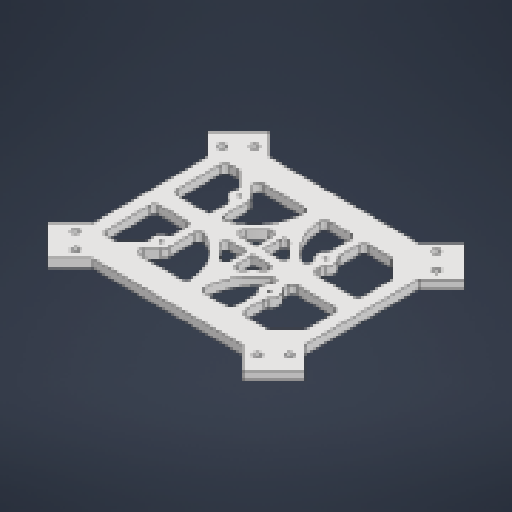
# Autodesk Inventor part: Base
Saved by Autodesk Inventor 2023 (Build 270158000, 158)
## iProperties
Created: 2023-01-21
Part Number: Base
Material: Generic
Document SubType Name: Modeling
Designer: Michael
Density: 1 g/cm^3
Appearance: Default
Author: Michael
Autodesk Inventor part; units mm, degrees
ref_plane "YZ Plane" through (0, 0, 0) normal (1, 0, 0) x (0, 1, 0)
ref_plane "XZ Plane" through (0, 0, 0) normal (0, 1, 0) x (-1, 0, 0)
ref_plane "XY Plane" through (0, 0, 0) normal (0, 0, 1) x (1, 0, 0)
sketch "Sketch1" plane through (0, 0, 0) normal (0, 1, 0) x (-1, 0, 0)
  line L0 (0, 0) -> (152.4, 0)
  line L1 (152.4, 0) -> (152.4, -127)
  line L2 (152.4, -127) -> (0, -127)
  line L3 (0, -127) -> (0, 0)
  circle A0 centre (10.775, -127.8974) radius 2.4765
  circle A1 centre (-0.8987, -116.2224) radius 2.4765
  circle A2 centre (-0.8987, -10.7776) radius 2.4765
  circle A3 centre (10.775, 0.8974) radius 2.4765
  line L4 (76.2, -127) -> (76.2, -50.8058)
  line L5 (152.4, -63.5) -> (91.8437, -63.5)
  line L6 (152.4, 0) -> (0, 0)
  circle A4 centre (10.775, 0.8974) radius 2.4765
  circle A5 centre (-0.8987, -10.7776) radius 2.4765
  line L7 (168.6133, -143.1442) -> (95.3909, -143.1442)
  line L8 (57.0091, -143.1442) -> (6.2091, -143.1442)
  circle A6 centre (153.2987, -10.7776) radius 2.4765
  circle A7 centre (141.625, 0.8974) radius 2.4765
  circle A8 centre (141.625, 0.8974) radius 2.4765
  circle A9 centre (153.2987, -10.7776) radius 2.4765
  line L9 (0, -127) -> (152.4, -127)
  circle A10 centre (-0.8987, -116.2224) radius 2.4765
  circle A11 centre (10.775, -127.8974) radius 2.4765
  circle A12 centre (10.775, -127.8974) radius 2.4765
  circle A13 centre (-0.8987, -116.2224) radius 2.4765
  line L10 (152.4, -127) -> (0, -127)
  line L11 (95.3909, -143.1442) -> (168.6133, -143.1442)
  line L12 (6.2091, -143.1442) -> (57.0091, -143.1442)
  line L13 (6.2832, 16.1645) -> (22.4494, 0)
  line L14 (22.4494, 0) -> (0, -22.4519)
  line L15 (0, -22.4519) -> (-16.1663, -6.2874)
  line L16 (-16.1663, -6.2874) -> (6.2832, 16.1645)
  line L17 (152.4, 0) -> (0, 0)
  line L18 (152.4, -127) -> (152.4, 0)
  circle A14 centre (153.2987, -10.7776) radius 2.4765
  circle A15 centre (141.625, 0.8974) radius 2.4765
  circle A16 centre (141.625, 0.8974) radius 2.4765
  circle A17 centre (153.2987, -10.7776) radius 2.4765
  line L19 (0, 0) -> (152.4, 0)
  line L20 (146.1168, 16.1645) -> (129.9506, 0)
  line L21 (129.9506, 0) -> (152.4, -22.4519)
  line L22 (152.4, -22.4519) -> (168.5663, -6.2874)
  line L23 (168.5663, -6.2874) -> (146.1168, 16.1645)
  line L24 (0, -127) -> (152.4, -127)
  circle A18 centre (-0.8987, -116.2224) radius 2.4765
  circle A19 centre (10.775, -127.8974) radius 2.4765
  circle A20 centre (10.775, -127.8974) radius 2.4765
  circle A21 centre (-0.8987, -116.2224) radius 2.4765
  line L25 (152.4, -127) -> (0, -127)
  circle A22 centre (153.2987, -116.2224) radius 2.4765
  circle A23 centre (153.2987, -116.2224) radius 2.4765
  circle A24 centre (141.625, -127.8974) radius 2.4765
  circle A25 centre (141.625, -127.8974) radius 2.4765
  line L26 (6.2832, -143.1645) -> (22.4494, -127)
  line L27 (22.4494, -127) -> (0, -104.5481)
  line L28 (0, -104.5481) -> (-16.1663, -120.7126)
  line L29 (-16.1663, -120.7126) -> (6.2832, -143.1645)
  line L30 (152.4, -127) -> (0, -127)
  line L31 (0, -127) -> (152.4, -127)
  circle A26 centre (153.2987, -116.2224) radius 2.4765
  circle A27 centre (141.625, -127.8974) radius 2.4765
  circle A28 centre (141.625, -127.8974) radius 2.4765
  circle A29 centre (153.2987, -116.2224) radius 2.4765
  line L32 (129.9506, -127) -> (152.4, -104.5481)
  line L33 (146.1168, -143.1645) -> (129.9506, -127)
  line L34 (152.4, -104.5481) -> (168.5663, -120.7126)
  line L35 (168.5663, -120.7126) -> (146.1168, -143.1645)
  point P0 (76.2, 0)
  point P1 (6.2628, -143.1442)
  point P2 (6.3035, -143.1442)
  point P3 (146.0965, -143.1442)
  point P4 (146.1372, -143.1442)
  dimension "d0" = 152.4
  constraints: 72 end point, 43 symmetric about line, 30 centre point, 4 horizontal, 2 midpoint, 2 parallel, 1 perpendicular, 1 vertical, 46 other
  measures "d0" distance of L1.end L2.end
extrude "Extrusion1" add sketch "Sketch1" along normal blind 6.35 contours L14 L3 A2 L0 A3 | L0 A3 L3 A2 L15 L16 L13 | L0 L21 L1 L32 L2 L27 L3 L14 | L20 L23 L22 L1 A6 L0 A7 | L0 A7 L1 A6 L21 | L27 L2 A0 L3 A1 | L3 A1 L2 A0 L26 L8 L29 L28 | L34 L35 L7 L33 L2 A24 L1 A22 | L1 A22 L2 A24 L32
sketch "Sketch11" plane through (0, 6.35, 0) normal (0, 1, 0) x (1, 0, 0)
  line L0 (-129.9506, 0) -> (-22.4494, 0) projected
  line L1 (-22.4494, 0) -> (-4.4879, -17.9595) projected
  line L2 (-4.4879, -17.9595) -> (17.9615, 4.4923) projected
  line L3 (17.9615, 4.4923) -> (0, 22.4519) projected
  line L4 (0, 22.4519) -> (0, 104.5481) projected
  line L5 (0, 104.5481) -> (17.9615, 122.5077) projected
  line L6 (17.9615, 122.5077) -> (-4.4879, 144.9595) projected
  line L7 (-4.4879, 144.9595) -> (-22.4494, 127) projected
  line L8 (-22.4494, 127) -> (-129.9506, 127) projected
  line L9 (-152.4, 104.5481) -> (-152.4, 22.4519) projected
  circle A0 centre (-10.775, -0.8974) radius 2.4765 projected
  circle A1 centre (0.8987, 10.7776) radius 2.4765 projected
  circle A2 centre (0.8987, 116.2224) radius 2.4765 projected
  circle A3 centre (-10.775, 127.8974) radius 2.4765 projected
  line L10 (-150.1188, 15.875) -> (-4.9505, 15.875)
  line L11 (-76.2, 0) -> (-76.2, 8.5621)
  line L12 (-22.4494, 127) -> (-129.9506, 127) projected
  line L13 (-79.375, 60.1756) -> (-104.775, 60.1756)
  line L14 (-79.375, 60.1756) -> (-79.375, 34.7756)
  arc A4 (-79.375, 34.7756) -> (-104.775, 60.1756) centre (-115.8345, 23.716) ccw
  line L15 (-74.8131, 59.9763) -> (-49.4131, 59.9763)
  line L16 (-74.8131, 59.9763) -> (-74.8131, 34.5763)
  arc A5 (-49.4131, 59.9763) -> (-74.8131, 34.5763) centre (-38.3536, 23.5168) ccw
  line L17 (-116.2036, 57.15) -> (-142.875, 57.15)
  line L18 (-82.272, 21.5362) -> (-82.272, 19.05)
  line L19 (-132.389, 19.05) -> (-142.875, 19.05)
  line L20 (-142.875, 19.05) -> (-142.875, 57.15)
  line L21 (-120.6293, 30.8097) -> (-132.389, 19.05)
  line L22 (-116.2036, 41.4682) -> (-116.2036, 57.15)
  line L23 (-82.272, 19.05) -> (-123.4088, 19.05)
  line L24 (-111.4454, 31.0134) -> (-123.4088, 19.05)
  line L25 (-111.4454, 31.0134) -> (-94.5266, 31.0134) construction
  arc A6 (-111.4454, 31.0134) -> (-109.8536, 35.3392) centre (-116.2025, 35.2196) ccw
  line L26 (-109.8536, 57.0906) -> (-109.8536, 35.3392)
  arc A7 (-82.272, 21.5362) -> (-109.8536, 57.0906) centre (-120.4848, 20.3679) ccw
  line L27 (-71.6381, 21.5362) -> (-71.6381, 18.6974)
  arc A8 (-49.4131, 55.641) -> (-71.6381, 21.5362) centre (-33.4125, 20.9198) ccw
  line L28 (-49.4131, 37.748) -> (-49.4131, 18.6974)
  line L29 (-43.0631, 37.6999) -> (-43.0631, 19.05)
  line L30 (-71.6381, 18.6974) -> (-49.4131, 18.6974)
  line L31 (-49.4131, 48.6912) -> (-49.4131, 55.641)
  arc A9 (-49.4131, 48.6912) -> (-49.4131, 37.748) centre (-46.2025, 43.2196) ccw
  arc A10 (-43.0631, 37.6999) -> (-43.0515, 48.7327) centre (-46.2025, 43.2196) ccw
  line L32 (-43.0631, 19.05) -> (-22.9954, 19.05)
  line L33 (-43.0515, 56.8024) -> (-9.525, 56.8024)
  line L34 (-43.0515, 48.7327) -> (-43.0515, 56.8024)
  line L35 (-9.525, 32.5204) -> (-9.525, 56.8024)
  line L36 (-22.9954, 19.05) -> (-9.525, 32.5204)
  line L37 (-22.9954, 19.05) -> (-3.9454, 19.05) construction
  line L38 (-129.9506, 127) -> (-147.9121, 144.9595) projected
  line L39 (-147.9121, 144.9595) -> (-170.3615, 122.5077) projected
  line L40 (-170.3615, 122.5077) -> (-152.4, 104.5481) projected
  line L41 (-152.4, 22.4519) -> (-170.3615, 4.4923) projected
  line L42 (-170.3615, 4.4923) -> (-147.9121, -17.9595) projected
  line L43 (-147.9121, -17.9595) -> (-129.9506, 0) projected
  line L44 (-76.2, 127) -> (-76.2, 0)
  line L45 (-129.9506, 0) -> (0, 0) projected
  line L46 (0, 63.5) -> (-152.4, 63.5)
  circle A11 centre (-46.2025, 43.2196) radius 1
  circle A12 centre (-116.2025, 35.2196) radius 1
  arc A13 (-116.2036, 41.4682) -> (-120.6293, 30.8097) centre (-116.2025, 35.2196) ccw
  line L47 (-22.9954, 107.95) -> (-3.9454, 107.95) construction
  line L48 (-76.2, 0) -> (-76.2, 127)
  line L49 (-79.375, 66.8244) -> (-104.775, 66.8244)
  line L50 (-79.375, 66.8244) -> (-79.375, 92.2244)
  arc A14 (-104.775, 66.8244) -> (-79.375, 92.2244) centre (-115.8345, 103.284) ccw
  arc A15 (-74.8131, 92.4237) -> (-49.4131, 67.0237) centre (-38.3536, 103.4832) ccw
  line L51 (-74.8131, 67.0237) -> (-74.8131, 92.4237)
  line L52 (-74.8131, 67.0237) -> (-49.4131, 67.0237)
  line L53 (-116.2036, 69.85) -> (-142.875, 69.85)
  line L54 (-82.272, 105.4638) -> (-82.272, 107.95)
  line L55 (-132.389, 107.95) -> (-142.875, 107.95)
  line L56 (-142.875, 107.95) -> (-142.875, 69.85)
  line L57 (-120.6293, 96.1903) -> (-132.389, 107.95)
  line L58 (-116.2036, 85.5318) -> (-116.2036, 69.85)
  line L59 (-82.272, 107.95) -> (-123.4088, 107.95)
  line L60 (-111.4454, 95.9866) -> (-123.4088, 107.95)
  line L61 (-111.4454, 95.9866) -> (-94.5266, 95.9866) construction
  arc A16 (-109.8536, 91.6608) -> (-111.4454, 95.9866) centre (-116.2025, 91.7804) ccw
  line L62 (-109.8536, 69.9094) -> (-109.8536, 91.6608)
  arc A17 (-109.8536, 69.9094) -> (-82.272, 105.4638) centre (-120.4848, 106.6321) ccw
  arc A18 (-71.6381, 105.4638) -> (-49.4131, 71.359) centre (-33.4125, 106.0802) ccw
  line L63 (-71.6381, 105.4638) -> (-71.6381, 108.3026)
  line L64 (-49.4131, 89.252) -> (-49.4131, 108.3026)
  line L65 (-43.0631, 89.3001) -> (-43.0631, 107.95)
  line L66 (-71.6381, 108.3026) -> (-49.4131, 108.3026)
  line L67 (-49.4131, 78.3088) -> (-49.4131, 71.359)
  arc A19 (-49.4131, 89.252) -> (-49.4131, 78.3088) centre (-46.2025, 83.7804) ccw
  arc A20 (-43.0515, 78.2673) -> (-43.0631, 89.3001) centre (-46.2025, 83.7804) ccw
  line L68 (-43.0631, 107.95) -> (-22.9954, 107.95)
  line L69 (-43.0515, 70.1976) -> (-9.525, 70.1976)
  line L70 (-43.0515, 78.2673) -> (-43.0515, 70.1976)
  line L71 (-9.525, 94.4796) -> (-9.525, 70.1976)
  line L72 (-22.9954, 107.95) -> (-9.525, 94.4796)
  circle A21 centre (-46.2025, 83.7804) radius 1
  circle A22 centre (-116.2025, 91.7804) radius 1
  arc A23 (-120.6293, 96.1903) -> (-116.2036, 85.5318) centre (-116.2025, 91.7804) ccw
  point P0 (-88.8938, 50.6568)
  point P1 (-102.8973, 47.4818)
  point P2 (-134.4732, 19.05)
  point P3 (-35.0401, 57.1784)
  point P4 (-43.0631, 28.375)
  point P5 (-49.4131, 28.2227)
  point P6 (-27.2644, 63.1524)
  point P7 (-110.1585, 36.9753)
  point P8 (-43.0515, 52.7675)
  point P9 (-88.8938, 76.3432)
  point P10 (-102.8973, 79.5182)
  point P11 (-35.0401, 69.8216)
  point P12 (-43.0631, 98.625)
  point P13 (-49.4131, 98.7773)
  point P14 (-43.0515, 74.2325)
  point P15 (-152.4, 0)
  point P16 (-13.0832, 0)
  point P17 (0, 13.0853)
  point P18 (0, 113.9147)
  point P19 (-13.0832, 127)
  point P20 (-152.4, 127)
  point P21 (-8.4668, 0)
  point P22 (0, 8.4699)
  point P23 (0, 118.5301)
  point P24 (-8.4668, 127)
  point P25 (-139.3168, 0)
  point P26 (0, 127)
  point P27 (-152.4, 8.4699)
  dimension "d109" = 15.875
  dimension "d121" = 25.4
  dimension "d122" = 25.4
  dimension "d123" = 38.1
  dimension "d127" = 3.175
  dimension "d130" = 3.175
  dimension "d131" = 135
  dimension "d133" = 6.35
  dimension "d141" = 3.175
  dimension "d146" = 0
  dimension "d147" = 6.35
  dimension "d150" = 6.35
  dimension "d151" = 3.175
  dimension "d152" = 45
  dimension "d153" = 19.05
  dimension "d156" = 6.344
  dimension "d157" = 6.35
  dimension "d159" = 25.4
  dimension "d160" = 25.4
  dimension "d161" = 38.1
  dimension "d164" = 6.9497
  dimension "d165" = 19.0506
  dimension "d166" = 3.175
  dimension "d167" = 1.3868
  dimension "d168" = 6.35
  dimension "d169" = 16.9188
  dimension "d174" = 6.35
  dimension "d176" = 9.525
  dimension "d177" = 9.525
  constraints: 110 end point, 50 symmetric about line, 33 point on circle, 24 centre point, 8 horizontal, 7 midpoint, 7 perpendicular, 5 vertical, 4 parallel, 4 point on line, 2 coincident, 2 concentric, 2 equal length, 14 other
  measures "d109" distance between parallel lines of L0 L10
  measures "d121" distance of L13.start L13.end
  measures "d122" distance of L13.start L14.end
  measures "d123" radius of A4
  measures "d127" distance between parallel lines of L19 L10
  measures "d130" vertical distance of point (-88.894, 50.657) point (-102.897, 47.482)
  measures "d131" angle of L24 L25
  measures "d133" distance between parallel lines of L21 L24
  measures "d141" distance between parallel lines of L10 L23
  measures "d146" distance from line of L31 L15.end
  measures "d147" horizontal distance of point (-43.063, 28.375) point (-49.413, 28.223)
  measures "d150" distance from line of point (-27.264, 63.152) L33
  measures "d151" distance between parallel lines of L10 L32
  measures "d152" angle of L37 L36
  measures "d153" distance of L32.end L35.start
  measures "d156" radius of A9
  measures "d157" radius of A10
  measures "d159" distance of L16.start L16.end
  measures "d160" distance of L16.start L15.end
  measures "d161" radius of A5
  measures "d164" distance of L31.start L31.end
  measures "d165" distance of L28.start L28.end
  measures "d166" distance between parallel lines of L44 L14
  measures "d167" distance between parallel lines of L44 L16
  measures "d168" radius of A6
  measures "d169" distance of L24.start L23.end
  measures "d174" distance between parallel lines of L26 L22
  measures "d176" distance between parallel lines of L9 L20
  measures "d177" distance between parallel lines of L4 L35
extrude "Extrusion12" cut sketch "Sketch11" against normal blind 17.4625 contours L14 A4 L13 | L15 A5 L16 | L22 A13 L21 L19 L20 L17 | L18 L23 L24 A6 L26 A7 | A8 L31 A9 L28 L30 L27 | A10 L34 L33 L35 L36 L32 L29 | A11 | A12 | L49 A14 L50 | A15 L52 L51 | L53 L56 L55 L57 A23 L58 | A17 L62 A16 L60 L59 L54 | L63 L66 L64 A19 L67 A18 | L65 L68 L72 L71 L69 L70 A20 | A21 | A22
fillet "Fillet2" radius 3.175 49 edges at (-142.875, 3.175, -19.05) (-142.875, 3.175, -57.15) (-116.2036, 3.175, -57.15) (-132.389, 3.175, -19.05) (-116.2036, 3.175, -41.4682) (-120.6293, 3.175, -30.8097) (-123.4088, 3.175, -19.05) (-109.8536, 3.175, -57.0906) (-82.272, 3.175, -19.05) (-104.775, 3.175, -60.1756) (-79.375, 3.175, -34.7756) (-74.8131, 3.175, -34.5763) (-49.4131, 3.175, -59.9763) (-71.6381, 3.175, -18.6974) (-49.4131, 3.175, -18.6974) (-49.4131, 3.175, -55.641) (-49.4131, 3.175, -37.748) (-49.4131, 3.175, -48.6912) (-43.0515, 3.175, -48.7327) (-43.0631, 3.175, -37.6999) (-43.0631, 3.175, -19.05) (-43.0515, 3.175, -56.8024) (-22.9954, 3.175, -19.05) (-9.525, 3.175, -32.5204) (-9.525, 3.175, -56.8024) (-132.389, 3.175, -107.95) (-22.9954, 3.175, -107.95) (-123.4088, 3.175, -107.95) (-142.875, 3.175, -107.95) (-109.8536, 3.175, -69.9094) (-142.875, 3.175, -69.85) (-104.775, 3.175, -66.8244) (-116.2036, 3.175, -85.5318) (-120.6293, 3.175, -96.1903) (-82.272, 3.175, -107.95) (-79.375, 3.175, -92.2244) (-49.4131, 3.175, -108.3026) (-74.8131, 3.175, -92.4237) (-49.4131, 3.175, -67.0237) (-49.4131, 3.175, -89.252) (-49.4131, 3.175, -78.3088) (-49.4131, 3.175, -71.359) (-71.6381, 3.175, -108.3026) (-43.0631, 3.175, -107.95) (-43.0631, 3.175, -89.3001) (-43.0515, 3.175, -78.2673) (-9.525, 3.175, -94.4796) (-43.0515, 3.175, -70.1976) (-9.525, 3.175, -70.1976)
body "Solid1"
